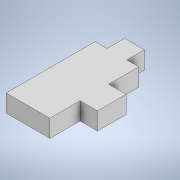
# Autodesk Inventor part: CotéV2
Saved by Autodesk Inventor 2020 (Build 240168000, 168)
## iProperties
Created: 2019-11-14
Part Number: CotéV2
Material: Générique
Document SubType Name: Modeling
Designer: erwan
Density: 1 g/cm^3
Appearance: Par défaut
Author: erwan
Autodesk Inventor part; units mm, degrees
ref_plane "YZ Plane" through (0, 0, 0) normal (1, 0, 0) x (0, 1, 0)
ref_plane "XZ Plane" through (0, 0, 0) normal (0, 1, 0) x (-1, 0, 0)
ref_plane "XY Plane" through (0, 0, 0) normal (0, 0, 1) x (1, 0, 0)
sketch "Esquisse1" plane through (0, 0, 0) normal (0, 1, 0) x (-1, 0, 0)
  line L0 (68.888, 27.0027) -> (13.888, 27.0027)
  line L1 (13.888, 27.0027) -> (13.888, -10.9973)
  line L2 (68.888, -62.9973) -> (68.888, 27.0027)
  line L3 (13.888, -10.9973) -> (-8.112, -10.9973)
  line L4 (-8.112, -10.9973) -> (-8.112, -46.9973)
  line L5 (-8.112, -46.9973) -> (13.888, -46.9973)
  line L6 (13.888, -46.9973) -> (13.888, -62.9973)
  line L7 (68.888, -62.9973) -> (68.888, -84.9973)
  line L8 (68.888, -84.9973) -> (53.888, -84.9973)
  line L9 (53.888, -84.9973) -> (53.888, -106.9973)
  line L10 (53.888, -106.9973) -> (28.888, -106.9973)
  line L11 (28.888, -106.9973) -> (28.888, -84.9973)
  line L12 (28.888, -84.9973) -> (13.888, -84.9973)
  line L13 (13.888, -84.9973) -> (13.888, -62.9973)
  point P0 (0, 0)
  dimension "d1" = 55
  dimension "d2" = 22
  dimension "d3" = 38
  dimension "d4" = 36
  dimension "d11" = 22
  dimension "d12" = 15
  dimension "d13" = 22
  dimension "d14" = 25
  constraints: 28 end point, 7 perpendicular, 4 horizontal, 3 parallel, 1 vertical
  measures "d1" distance between parallel lines of L1 L2
  measures "d2" distance between parallel lines of L4 L1
  measures "d3" distance between parallel lines of L0 L3
  measures "d4" distance between parallel lines of L3 L5
  measures "d11" distance of L2.start L7.end
  measures "d12" distance of L7.end L8.end
  measures "d13" distance of L8.end L9.end
  measures "d14" distance of L9.end L10.end
extrude "Extrusion1" add sketch "Esquisse1" along normal blind 22
